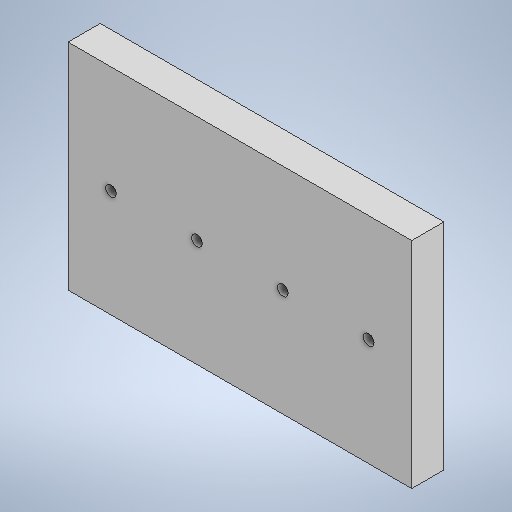
# Autodesk Inventor part: Part_Back
Saved by Autodesk Inventor 2025 (Build 290162010, 162A)
## iProperties
Created: 2024-07-05
Part Number: Part_Back
Material: Generic
Document SubType Name: Modeling
Designer: kani2
Density: 1 g/cm^3
Appearance: Default
Author: kani2
Autodesk Inventor part; units mm, degrees
ref_plane "YZ Plane" through (0, 0, 0) normal (1, 0, 0) x (0, 1, 0)
ref_plane "XZ Plane" through (0, 0, 0) normal (0, 1, 0) x (-1, 0, 0)
ref_plane "XY Plane" through (0, 0, 0) normal (0, 0, 1) x (1, 0, 0)
sketch "Sketch1" plane through (0, 0, 0) normal (0, 0, 1) x (1, 0, 0)
  line L0 (-101.6, 63.5) -> (101.6, 63.5)
  line L1 (101.6, 63.5) -> (101.6, -63.5)
  line L2 (101.6, -63.5) -> (-101.6, -63.5)
  line L3 (-101.6, -63.5) -> (-101.6, 63.5)
  line L4 (-101.6, 63.5) -> (101.6, -63.5) construction
  line L5 (101.6, 63.5) -> (-101.6, -63.5) construction
  circle A0 centre (-76.2, 0) radius 3.175
  circle A1 centre (-25.4, 0) radius 3.175
  circle A2 centre (25.4, 0) radius 3.175
  circle A3 centre (76.2, 0) radius 3.175
  point P0 (0, 0)
  dimension "d0" = 203.2
  dimension "d1" = 127
  dimension "d2" = 6.35
  dimension "d3" = 6.35
  dimension "d4" = 6.35
  dimension "d5" = 6.35
  dimension "d6" = 25.4
  dimension "d7" = 76.2
  dimension "d8" = 127
  dimension "d9" = 177.8
  constraints: 12 end point, 4 centre point, 2 midpoint, 2 parallel, 1 horizontal, 1 perpendicular
  measures "d0" distance of L1.end L2.end
  measures "d1" distance of L0.end L1.end
  measures "d2" diameter of A0
  measures "d3" diameter of A1
  measures "d4" diameter of A2
  measures "d5" diameter of A3
  measures "d6" distance from line of L3 A0.centre
  measures "d7" distance from line of L3 A1.centre
  measures "d8" distance from line of L3 A2.centre
  measures "d9" distance from line of L3 A3.centre
extrude "Extrusion1" add sketch "Sketch1" along normal blind 19.05 contours L0 L1 L2 L3 | A0 | A1 | A2 | A3
sketch "Sketch2" plane through (0, 0, 0) normal (0, 0, -1) x (-1, 0, 0)
  circle A0 centre (-76.2, 0) radius 3.175
  circle A1 centre (-25.4, 0) radius 3.175
  circle A2 centre (25.4, 0) radius 3.175
  circle A3 centre (76.2, 0) radius 3.175
  line L0 (-101.6, 63.5) -> (101.6, 63.5) projected
  line L1 (-101.6, -63.5) -> (-101.6, 63.5) projected
  point P0 (0, 0)
  dimension "d12" = 6.35
  dimension "d13" = 6.35
  dimension "d14" = 6.35
  dimension "d15" = 6.35
  dimension "d17" = 63.5
  dimension "d18" = 63.5
  dimension "d19" = 25.4
  dimension "d20" = 76.2
  dimension "d21" = 127
  dimension "d22" = 177.8
  constraints: 4 centre point
  measures "d12" diameter of A0
  measures "d13" diameter of A1
  measures "d14" diameter of A2
  measures "d15" diameter of A3
  measures "d17" distance from line of L0 A0.centre
  measures "d18" distance from line of L0 A1.centre
  measures "d19" distance from line of L1 A0.centre
  measures "d20" distance from line of L1 A1.centre
  measures "d21" distance from line of L1 A2.centre
  measures "d22" distance from line of L1 A3.centre
extrude "Extrusion2" cut sketch "Sketch2" against normal blind 19.05
body "Solid1"
